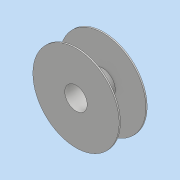
# Autodesk Inventor part: szpula
Saved by Autodesk Inventor 2017 (Build 210142000, 142)
## iProperties
Created: 2017-11-03
Part Number: szpula
Material: Ogólny
Document SubType Name: Modeling
Designer: Kuba01
Density: 1 g/cm^3
Appearance: Domyślna
Author: Kuba01
Autodesk Inventor part; units mm, degrees
ref_plane "YZ Plane" through (0, 0, 0) normal (1, 0, 0) x (0, 1, 0)
ref_plane "XZ Plane" through (0, 0, 0) normal (0, 1, 0) x (-1, 0, 0)
ref_plane "XY Plane" through (0, 0, 0) normal (0, 0, 1) x (1, 0, 0)
sketch "Szkic1" plane through (0, 0, 0) normal (0, 0, 1) x (1, 0, 0)
  line L0 (10.5195, 87.461) -> (10.5195, -76.7273)
  line L1 (-15.4805, 77.7078) -> (-89.4805, 77.7078)
  line L2 (-89.4805, 77.7078) -> (-89.4805, 74.7078)
  line L3 (-89.4805, 74.7078) -> (-18.4805, 74.7078)
  line L4 (-18.4805, 74.7078) -> (-18.4805, 15.7078)
  line L5 (-18.4805, 15.7078) -> (-89.4805, 15.7078)
  line L6 (-89.4805, 15.7078) -> (-89.4805, 12.7078)
  line L7 (-89.4805, 12.7078) -> (-15.4805, 12.7078)
  line L8 (-15.4805, 77.7078) -> (-15.4805, 12.7078)
  point P0 (0, 0)
  dimension "d0" = 65
  dimension "d1" = 52
  dimension "d2" = 58
  dimension "d3" = 3
  dimension "d4" = 3
  dimension "d5" = 200
  constraints: 18 end point, 6 perpendicular, 2 point on line, 1 horizontal, 1 vertical
  measures "d0" distance between parallel lines of L7 L1
  measures "d1" diameter of L8 L0
  measures "d2" diameter of L4 L0
  measures "d3" distance between parallel lines of L1 L3
  measures "d4" distance between parallel lines of L5 L7
  measures "d5" diameter of L2 L0
revolve "Obrót1" add sketch "Szkic1" angle 360 about axis through (10.5195, 87.461, 0) along (0, -1, 0)
